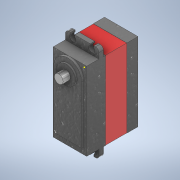
# Autodesk Inventor part: serwo 30x70
Saved by Autodesk Inventor 2021 (Build 250183000, 183)
## iProperties
Created: 2021-10-25
Part Number: serwo 30x70
Material: Generic
Document SubType Name: Modeling
Designer: Łukasz
Density: 1 g/cm^3
Appearance: Default
Author: Łukasz
Autodesk Inventor part; units mm, degrees
ref_plane "YZ Plane" through (0, 0, 0) normal (1, 0, 0) x (0, 1, 0)
ref_plane "XZ Plane" through (0, 0, 0) normal (0, 1, 0) x (-1, 0, 0)
sketch "Sketch1" plane through (0, 0, 0) normal (0, 0, 1) x (1, 0, 0)
  line L0 (0, 0) -> (-30, 0)
  line L1 (-30, 0) -> (-30, -70)
  line L2 (-30, -70) -> (0, -70)
  line L3 (0, -70) -> (0, 0)
  dimension "d0" = 30
  dimension "d1" = 70
  constraints: 8 end point, 2 parallel, 1 horizontal, 1 perpendicular
  measures "d0" distance of L2.end L1.end
  measures "d1" distance of L1.end L0.end
extrude "Extrusion1" add sketch "Sketch1" along normal blind 10
sketch "Sketch2" plane through (0, 0, 10) normal (0, 0, 1) x (1, 0, 0)
  line L0 (-30, 0) -> (-30, -70) projected
  line L1 (-30, -70) -> (0, -70) projected
  line L2 (0, -70) -> (0, 0) projected
  line L3 (0, 0) -> (-30, 0) projected
  line L4 (0, 0) -> (-30, 0) projected
  line L5 (-30, -70) -> (0, -70) projected
  line L6 (-0.1, -70) -> (-0.1, -0.1)
  line L7 (-0.1, -0.1) -> (-30, -0.1)
  line L8 (-29.9, 0) -> (-29.9, -70)
  line L9 (-30, -69.9) -> (0, -69.9)
  point P0 (-29.9, -69.9)
  point P1 (-0.1, -69.9)
  point P2 (-29.9, -0.1)
  dimension "d29" = 0.1
  dimension "d30" = 0.1
  dimension "d31" = 0.1
  constraints: 8 end point, 2 parallel, 1 other
  measures "d29" distance between parallel lines of L2 L6
  measures "d30" distance between parallel lines of L0 L8
  measures "d31" distance between parallel lines of L1 L9
extrude "Extrusion2" add sketch "Sketch2" along normal blind 19 contours L7 L6 L9 L8
sketch "Sketch3" plane through (0, 0, 29) normal (0, 0, 1) x (1, 0, 0)
  line L0 (-30, -70) -> (0, -70) projected
  line L1 (-30, 0) -> (-30, -70) projected
  line L2 (0, -70) -> (0, 0) projected
  line L3 (-30, -70) -> (0, -70) projected
  line L4 (0, 0) -> (-30, 0) projected
  line L5 (0, 0) -> (-30, 0) projected
  line L6 (0, -70) -> (0, 0) projected
  point P0 (-0.01, -70)
  point P1 (-0.01, 0)
extrude "Extrusion3" add sketch "Sketch3" along normal blind 19
sketch "Sketch4" plane through (0, 0, 48) normal (0, 0, 1) x (1, 0, 0)
  circle A0 centre (-15, -12.5) radius 8.5
  line L0 (0, 0) -> (-30, 0) projected
  dimension "d8" = 17
  dimension "d26" = 12.5
  constraints: 1 centre point
  measures "d8" diameter of A0
  measures "d26" distance from line of L0 A0.centre
extrude "Extrusion4" add sketch "Sketch4" along normal blind 1.5
sketch "Sketch5" plane through (-15, -12.5, 49.5) normal (0, 0, 1) x (1, 0, 0)
  circle A0 centre (0, 0) radius 3.9
  point P0 (15, 12.5)
  dimension "d11" = 7.8
  constraints: 1 centre point
  measures "d11" diameter of A0
extrude "Extrusion5" add sketch "Sketch5" along normal blind 6.5
ref_plane "Work Plane1" through (0, 0, 31) normal (0, 0, 1) x (1, 0, 0)
sketch "Sketch6" plane through (0, 0, 31) normal (0, 0, 1) x (1, 0, 0)
  line L0 (-30, -70) -> (0, -70) projected
  line L1 (0, -70) -> (-30, -70)
  line L2 (-30, -70) -> (-30, -78)
  line L3 (0, -78) -> (0, -70)
  arc A0 (-4.6303, -76.5166) -> (-7.7916, -76.9278) centre (-6.5, -74.5) ccw
  arc A1 (-21.6303, -76.5166) -> (-25.3697, -76.5166) centre (-23.5, -74.5) ccw
  line L4 (-4.6303, -76.5166) -> (-4.6303, -78)
  line L5 (-7.7916, -76.9278) -> (-7.7916, -78)
  line L6 (-4.6303, -78) -> (0, -78)
  line L7 (-30, -78) -> (-25.3697, -78)
  line L8 (-21.6303, -78) -> (-7.7916, -78)
  line L9 (-21.6303, -76.5166) -> (-21.6303, -78)
  line L10 (-25.3697, -76.5166) -> (-25.3697, -78)
  line L11 (0, -70) -> (0, 0) projected
  line L12 (0, -35) -> (-30, -35) construction
  line L13 (-30, 0) -> (0, 0)
  line L14 (0, 0) -> (-30, 0)
  line L15 (-30, 0) -> (-30, 8)
  line L16 (0, 8) -> (0, 0)
  arc A2 (-7.7916, 6.9278) -> (-4.6303, 6.5166) centre (-6.5, 4.5) ccw
  arc A3 (-25.3697, 6.5166) -> (-21.6303, 6.5166) centre (-23.5, 4.5) ccw
  line L17 (-4.6303, 6.5166) -> (-4.6303, 8)
  line L18 (-7.7916, 6.9278) -> (-7.7916, 8)
  line L19 (-4.6303, 8) -> (0, 8)
  line L20 (-30, 8) -> (-25.3697, 8)
  line L21 (-21.6303, 8) -> (-7.7916, 8)
  line L22 (-21.6303, 6.5166) -> (-21.6303, 8)
  line L23 (-25.3697, 6.5166) -> (-25.3697, 8)
  point P0 (-0.01, -70)
  dimension "d15" = 30
  dimension "d16" = 8
  dimension "d17" = 5.5
  dimension "d18" = 5.5
  dimension "d21" = 6.5
  dimension "d22" = 6.5
  constraints: 44 end point, 14 symmetric about line, 9 perpendicular, 8 point on circle, 4 centre point, 4 parallel, 2 horizontal, 1 midpoint, 2 other
  measures "d15" distance of L3.start L2.end
  measures "d16" distance of L2.end L1.end
  measures "d17" diameter of A0
  measures "d18" diameter of A1
  measures "d21" distance from line of L2 A1.centre
  measures "d22" distance from line of L3 A0.centre
extrude "Extrusion6" add sketch "Sketch6" along normal blind 4
fillet "Fillet1" radius 3 4 edges at (-30, 8, 33) (0, 8, 33) (-30, -78, 33) (0, -78, 33)
sketch "Sketch7" plane through (0, 0, 48) normal (0, 0, 1) x (1, 0, 0)
  point P0 (0, 0)
sketch "Sketch8" plane through (0, 0, 48) normal (0, 0, 1) x (1, 0, 0)
  circle A0 centre (-15, -12.5) radius 8.5 projected
  circle A1 centre (-15, -12.5) radius 12.5
  line L0 (0, -70) -> (0, 0) projected
  line L1 (-2.5, -64) -> (-27.5, -64)
  line L2 (-30, 0) -> (-30, -70) projected
  line L3 (-2.5, -12.5) -> (-2.5, -64)
  line L4 (-27.5, -12.5) -> (-27.5, -64)
  line L5 (-30, -70) -> (0, -70) projected
  line L6 (0, 0) -> (-30, 0) projected
  point P0 (-15, 0)
  constraints: 6 end point, 2 perpendicular, 2 point on circle, 2 tangent, 1 centre point, 1 coincident, 1 horizontal
extrude "Extrusion7" cut sketch "Sketch8" against normal blind 2 contours L6 L0 L5 L2
body "Solid1"
